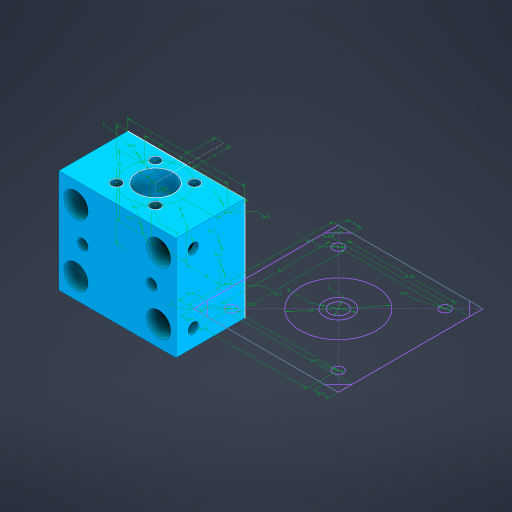
# Autodesk Inventor part: ZX Axis Carriage
Saved by Autodesk Inventor 2024.2 (Build 282272000, 272)
## iProperties
Created: 2024-10-02
Part Number: ZX Axis Carriage
Material: Generic
Document SubType Name: Modeling
Designer: jerem
Density: 1 g/cm^3
Appearance: Default
Author: jerem
Autodesk Inventor part; units mm, degrees
ref_plane "YZ Plane" through (0, 0, 0) normal (1, 0, 0) x (0, 1, 0)
ref_plane "XZ Plane" through (0, 0, 0) normal (0, 1, 0) x (-1, 0, 0)
ref_plane "XY Plane" through (0, 0, 0) normal (0, 0, 1) x (1, 0, 0)
sketch "Sketch1" plane through (0, 0, 0) normal (0, 0, 1) x (1, 0, 0)
  circle A0 centre (-12, 9) radius 1.5
  line L0 (12, -9) -> (-12, -9) construction
  line L1 (-12, -9) -> (-12, 9) construction
  line L2 (-12, 9) -> (12, 9) construction
  line L3 (12, 9) -> (12, -9) construction
  line L4 (12, -9) -> (-12, 9) construction
  line L5 (-12, -9) -> (12, 9) construction
  circle A1 centre (12, 9) radius 1.5
  circle A2 centre (12, -9) radius 1.5
  circle A3 centre (-12, -9) radius 1.5
  line L6 (17, -15) -> (-17, -15)
  line L7 (-17, -15) -> (-17, 15)
  line L8 (-17, 15) -> (17, 15)
  line L9 (17, 15) -> (17, -15)
  line L10 (17, -15) -> (-17, 15) construction
  line L11 (-17, -15) -> (17, 15) construction
  circle A4 centre (0, 0) radius 4
  circle A5 centre (12, 9) radius 3.5
  circle A6 centre (-12, 9) radius 3.5
  circle A7 centre (-12, -9) radius 3.5
  circle A8 centre (12, -9) radius 3.5
  circle A9 centre (10, 0) radius 1.5
  circle A10 centre (-10, 0) radius 1.5
  line L12 (10, 0) -> (0, 0) construction
  line L13 (0, 0) -> (-10, 0) construction
  point P0 (0, 0)
  dimension "d0" = 3
  dimension "d1" = 24
  dimension "d2" = 18
  dimension "d3" = 3
  dimension "d4" = 3
  dimension "d5" = 3
  dimension "d6" = 34
  dimension "d7" = 30
  dimension "d8" = 8
  dimension "d15" = 2
  dimension "d16" = 2
  dimension "d17" = 2
  dimension "d18" = 2
  dimension "d59" = 3
  dimension "d60" = 10
  dimension "d61" = 10
  dimension "d62" = 3
  constraints: 28 end point, 11 centre point, 11 coincident, 5 equal length, 4 midpoint, 3 horizontal, 2 perpendicular
  measures "d0" diameter of A0
  measures "d1" distance of L4.end L3.start
  measures "d2" distance of L0.end L4.end
  measures "d3" diameter of A3
  measures "d4" diameter of A1
  measures "d5" diameter of A2
  measures "d6" distance of L7.end L8.end
  measures "d7" distance of L6.end L7.end
  measures "d8" diameter of A4
  measures "d15" radial gap between concentric circles of A5 A1
  measures "d16" radial gap between concentric circles of A6 A0
  measures "d17" radial gap between concentric circles of A7 A3
  measures "d18" radial gap between concentric circles of A8 A2
  measures "d59" diameter of A9
  measures "d60" distance of L12.end L12.start
  measures "d61" distance of L12.end L13.end
  measures "d62" diameter of A10
extrude "Extrusion1" add sketch "Sketch1" along normal blind 20 contours L6 L7 L8 L9 | A4
extrude "Extrusion3" add sketch "Sketch1" along normal blind 5 from surface at 0 contours A5 | A6 | A7 | A8
sketch "Sketch2" plane through (-17, 15, 0) normal (0, 1, 0) x (1, 0, 0)
  circle A0 centre (17, -9) radius 5.3
  line L0 (17, -9) -> (17, 0) construction
  line L1 (17, -9) -> (22.6569, -14.6569) construction
  line L2 (17, -9) -> (25, -9) construction
  circle A1 centre (22.6569, -14.6569) radius 1.5
  circle A2 centre (22.6569, -3.3431) radius 1.5
  circle A3 centre (11.3431, -3.3431) radius 1.5
  circle A4 centre (11.3431, -14.6569) radius 1.5
  line L3 (17, -9) -> (17, 11) construction
  line L4 (20.5261, 0) -> (13.5408, 0) construction
  dimension "d11" = 10.6
  dimension "d12" = 9
  dimension "d21" = 45
  dimension "d22" = 8
  dimension "d23" = 3
  dimension "d26" = 360
  dimension "d49" = 20
  dimension "d50" = 11
  constraints: 10 end point, 5 centre point, 2 horizontal, 1 coincident, 1 equal length, 1 perpendicular, 1 point on line, 1 vertical, 9 other
  measures "d11" diameter of A0
  measures "d12" distance of L0.start L0.end
  measures "d21" angle of L1 L2
  measures "d22" distance of L0.start L1.end
  measures "d23" diameter of A1
  measures "d49" distance of L0.start L3.end
  measures "d50" distance from line of L3.end L4
extrude "Extrusion2" cut sketch "Sketch2" against normal through all contours A0
extrude "Extrusion4" cut sketch "Sketch2" against normal blind 10 contours A1 | A2 | A3 | A4
sketch "Sketch3" plane through (0, 0, 0) normal (0, 1, 0) x (-1, 0, 0)
  line L0 (-64.168, -21.8863) -> (-22.168, -21.8863)
  line L1 (-22.168, -21.8863) -> (-22.168, 20.1137)
  line L2 (-22.168, 20.1137) -> (-64.168, 20.1137)
  line L3 (-64.168, 20.1137) -> (-64.168, -21.8863)
  line L4 (-64.168, -21.8863) -> (-22.168, 20.1137) construction
  line L5 (-22.168, -21.8863) -> (-64.168, 20.1137) construction
  circle A0 centre (-27.668, 14.6137) radius 1.5
  circle A1 centre (-27.668, -16.3863) radius 1.5
  circle A2 centre (-58.668, -16.3862) radius 1.5
  circle A3 centre (-58.668, 14.6138) radius 1.5
  circle A4 centre (-43.168, -0.8863) radius 11
  circle A5 centre (-43.168, -0.8863) radius 4
  line L6 (-22.168, -17.8863) -> (-26.168, -21.8863)
  line L7 (-22.168, 16.1137) -> (-26.168, 20.1137)
  line L8 (-60.168, -21.8863) -> (-64.168, -17.8863)
  line L9 (-64.168, 16.1137) -> (-60.168, 20.1137)
  circle A6 centre (-43.168, -0.8863) radius 2.5
  point P0 (0, 0)
  dimension "d30" = 42
  dimension "d31" = 31
  dimension "d32" = 31
  dimension "d33" = 31
  dimension "d34" = 31
  dimension "d35" = 3
  dimension "d36" = 3
  dimension "d37" = 3
  dimension "d38" = 3
  dimension "d39" = 22
  dimension "d40" = 8
  dimension "d41" = 4
  dimension "d42" = 4
  dimension "d43" = 4
  dimension "d44" = 4
  dimension "d45" = 4
  dimension "d46" = 4
  dimension "d47" = 4
  dimension "d48" = 5
  constraints: 20 end point, 11 point on line, 7 centre point, 4 perpendicular, 3 coincident, 2 midpoint, 2 parallel, 1 horizontal
  measures "d30" distance of L0.end L2.start
  measures "d31" distance of A1.centre A0.centre
  measures "d32" distance of A2.centre A1.centre
  measures "d33" distance of A3.centre A2.centre
  measures "d34" distance of A0.centre A3.centre
  measures "d35" diameter of A0
  measures "d36" diameter of A1
  measures "d37" diameter of A2
  measures "d38" diameter of A3
  measures "d39" diameter of A4
  measures "d40" diameter of A5
  measures "d41" distance of L0.end L6.end
  measures "d42" distance of L0.end L6.start
  measures "d43" distance of L2.start L7.end
  measures "d44" distance of L7.start L2.start
  measures "d45" distance of L3.start L9.end
  measures "d46" distance of L3.start L9.start
  measures "d47" distance of L0.start L8.end
  measures "d48" diameter of A6
sketch "Sketch4" plane through (17, -15, 0) normal (1, 0, 0) x (0, 0, -1)
  circle A0 centre (-15, 25) radius 1.5
  line L0 (-20, 0) -> (-20, 30) projected
  line L1 (0, 30) -> (-20, 30) projected
  circle A1 centre (-15, 5) radius 1.5
  line L2 (0, 0) -> (-20, 0) projected
  point P0 (0, 15)
  dimension "d51" = 3
  dimension "d52" = 5
  dimension "d53" = 5
  dimension "d54" = 3
  dimension "d55" = 5
  dimension "d56" = 5
  constraints: 2 centre point
  measures "d51" diameter of A0
  measures "d52" distance from line of L0 A0.centre
  measures "d53" distance from line of L1 A0.centre
  measures "d54" diameter of A1
  measures "d55" distance from line of L0 A1.centre
  measures "d56" distance from line of L2 A1.centre
extrude "Extrusion5" cut sketch "Sketch4" against normal blind 5
equation "\"d3\" = d0"
equation "\"d4\" = d0"
equation "\"d5\" = d0"
equation "\"d16\" = d15"
equation "\"d17\" = d15"
equation "\"d18\" = d15"
equation "\"d61\" = d60"
equation "\"d32\" = d31"
equation "\"d33\" = d31"
equation "\"d34\" = d31"
equation "\"d36\" = d35"
equation "\"d37\" = d35"
equation "\"d38\" = d35"
equation "\"d42\" = d41"
equation "\"d43\" = d41"
equation "\"d44\" = d41"
equation "\"d45\" = d41"
equation "\"d46\" = d41"
equation "\"d47\" = d41"
equation "\"d54\" = d51"
equation "\"d55\" = d52"
equation "\"d56\" = d53"
body "Solid1"
